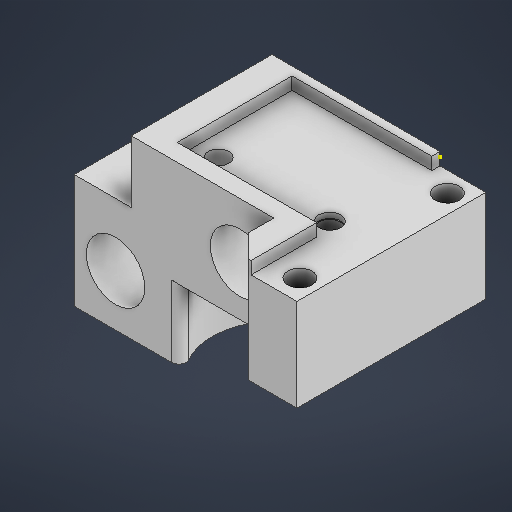
# Autodesk Inventor part: 固定传动
Saved by Autodesk Inventor 2025 (Build 290162000, 162)
## iProperties
Created: 2025-12-09
Part Number: 固定传动
Material: 常规
Document SubType Name: Modeling
Designer: XH
Density: 1 g/cm^3
Appearance: 默认
Author: XH
Autodesk Inventor part; units mm, degrees
ref_plane "YZ Plane" through (0, 0, 0) normal (1, 0, 0) x (0, 1, 0)
ref_plane "XZ Plane" through (0, 0, 0) normal (0, 1, 0) x (-1, 0, 0)
ref_plane "XY Plane" through (0, 0, 0) normal (0, 0, 1) x (1, 0, 0)
sketch "草图1" plane through (0, 0, 0) normal (0, 0, 1) x (1, 0, 0)
  line L0 (-22.2679, -12.5636) -> (3.7321, -12.5636) projected
  line L1 (-24.2679, 7.4364) -> (5.7321, 7.4364)
  line L2 (5.7321, 7.4364) -> (5.7321, -12.5636)
  line L3 (5.7321, -12.5636) -> (-24.2679, -12.5636)
  line L4 (-24.2679, -12.5636) -> (-24.2679, 7.4364)
  point P0 (-22.2679, -12.5636)
  point P1 (3.7321, -12.5636)
  dimension "d4" = 30
  dimension "d5" = 20
  constraints: 8 end point, 2 parallel, 1 collinear, 1 horizontal, 1 perpendicular
  measures "d4" distance of L1.start L1.end
  measures "d5" distance of L1.end L2.end
extrude "拉伸1" add sketch "草图1" along normal blind 19
sketch "草图2" plane through (0, 0, 0) normal (0, 0, -1) x (-1, 0, 0)
  line L0 (24.2679, 7.4364) -> (24.2679, -12.5636) projected
  line L1 (24.2679, -12.5636) -> (31.2679, -12.5636)
  line L2 (31.2679, -12.5636) -> (31.2679, -0.5636)
  line L3 (31.2679, -0.5636) -> (24.2679, -0.5636)
  line L4 (24.2679, -0.5636) -> (24.2679, -12.5636)
  point P0 (0, 0)
  dimension "d6" = 7
  dimension "d7" = 12
  constraints: 8 end point, 2 parallel, 1 horizontal, 1 perpendicular
  measures "d6" distance of L2.end L3.end
  measures "d7" distance of L1.end L2.end
extrude "拉伸2" add sketch "草图2" against normal up to surface (19 mm away)
sketch "草图3" plane through (0, 0, 0) normal (0, 0, -1) x (-1, 0, 0)
  circle A0 centre (-0.6256, 1.5535) radius 3
  circle A1 centre (26.4728, -5.3671) radius 4.1
  point P0 (0, 0)
  dimension "d10" = 6
  dimension "d11" = 8.2
  constraints: 2 centre point
  measures "d10" diameter of A0
  measures "d11" diameter of A1
extrude "拉伸3" cut sketch "草图3" against normal blind 40
sketch "草图4" plane through (5.7321, -12.5636, 0) normal (1, 0, 0) x (0, 0, -1)
  line L0 (-19, 0) -> (-4, 0)
  line L1 (-4, 0) -> (-4, 10)
  line L2 (-4, 10) -> (-19, 10)
  line L3 (-19, 10) -> (-19, 0)
  point P0 (0, 12.5636)
  dimension "d14" = 10
  dimension "d15" = 15
  constraints: 8 end point, 2 parallel, 1 horizontal, 1 perpendicular
  measures "d14" distance of L2.end L0.start
  measures "d15" distance of L1.end L2.end
extrude "拉伸4" cut sketch "草图4" against normal blind 21.75
chamfer "倒角1" distance 4 angle 45 1 edges at (-24.2679, -0.5636, 9.5)
sketch "草图5" plane through (5.7321, -12.5636, 0) normal (1, 0, 0) x (0, 0, -1)
  line L0 (-4, 0) -> (-19, 0) projected
  line L1 (-4, 0) -> (0, 0)
  line L2 (0, 0) -> (0, 10)
  line L3 (0, 10) -> (-4, 10)
  line L4 (-4, 10) -> (-4, 0)
  line L5 (0, 0) -> (0, 20) projected
  line L6 (-19, 10) -> (-4, 10) projected
  point P0 (0, 12.5636)
  constraints: 8 end point, 2 collinear, 2 parallel, 1 horizontal, 1 perpendicular
extrude "拉伸5" cut sketch "草图5" against normal blind 10
sketch "草图6" plane through (5.7321, -2.5636, 0) normal (0, -1, 0) x (1, 0, 0)
  line L0 (0, 0) -> (0, 19) projected
  line L1 (0, 0) -> (-8, 0)
  line L2 (-8, 0) -> (-8, 25.7509)
  line L3 (-8, 25.7509) -> (0, 25.7509)
  line L4 (0, 25.7509) -> (0, 0)
  line L5 (-12.3, 25.7509) -> (0, 25.7509) projected
  line L6 (-21.75, 19) -> (0, 19) projected
  line L7 (-8, 25.7509) -> (-10, 25.7509)
  line L8 (-10, 25.7509) -> (-10, 19)
  line L9 (-10, 19) -> (-8, 19)
  line L10 (-8, 19) -> (-8, 25.7509)
  point P0 (-5.7321, 0)
  point P1 (-8, 19)
  dimension "d23" = 8
  dimension "d28" = 10
  constraints: 16 end point, 4 parallel, 2 horizontal, 2 perpendicular, 1 collinear, 1 point on line
  measures "d23" distance between parallel lines of L2 L4
  measures "d28" distance between parallel lines of L4 L8
extrude "拉伸6" add sketch "草图6" against normal up to surface (10 mm away)
sketch "草图8" plane through (0, 0, 0) normal (0, 0, -1) x (-1, 0, 0)
  circle A0 centre (-0.6256, 1.5535) radius 3
  point P0 (0, 0)
  constraints: 1 centre point, 2 other
extrude "拉伸7" cut sketch "草图8" against normal blind 42.75
fillet "圆角1" radius 4 1 edges at (-4.2679, 2.4364, 19)
sketch "草图9" plane through (0, 0, 0) normal (0, 0, -1) x (-1, 0, 0)
  circle A0 centre (9.0791, 4.3462) radius 4.1
  point P0 (0, 0)
  dimension "d35" = 8.2
  constraints: 1 centre point, 1 other
  measures "d35" diameter of A0
extrude "拉伸8" cut sketch "草图9" against normal blind 33.75
delete faces "删除1" heal yes whole lump no faces at (-4.5364, 0.7697, 21.5592)
delete faces "删除2" heal yes whole lump no faces at (-1.434, 3.7348, 17.1673)
offset faces "大小1" outward 3 faces at (2.3988, 7.4364, 14.917) (-15.9384, 7.4364, 6.3333)
sketch "草图10" plane through (-16.0179, -2.5636, 19) normal (0, -1, 0) x (1, 0, 0)
  ellipse E0 centre (19.1097, 3.7017) end of major axis (18.1097, 3.7017) minor radius 1 projected
  ellipse E1 centre (19.1586, -16.9435) end of major axis (18.1586, -16.9435) minor radius 1 projected
  circle A0 centre (19.1097, 3.7017) radius 1.7
  circle A1 centre (19.1586, -16.9435) radius 1.7
  point P0 (16.0179, -19)
  dimension "d57" = 3.4
  dimension "d58" = 3.4
  constraints: 2 centre point, 2 coincident, 2 other
  measures "d57" diameter of A0
  measures "d58" diameter of A1
extrude "拉伸9" cut sketch "草图10" against normal blind 33.75 contours E0 | E1 | A0 | A1
offset faces "大小2" outward 1 faces at (-31.2679, -8.5636, 6.3333)
offset faces "大小3" outward 4 faces at (-30.9346, -0.5636, 6.3333)
sketch "草图11" plane through (-4.2679, -2.5636, 25.7509) normal (0, 0, 1) x (1, 0, 0)
  line L0 (10, 13) -> (-20, 13) projected
  line L1 (10, 13) -> (-20.4657, 13)
  line L2 (-20.4657, 13) -> (-20.4657, 12.2117)
  line L3 (-20.4657, 12.2117) -> (10, 12.2117)
  line L4 (10, 12.2117) -> (10, 13)
  line L5 (-8.462, 12.203) -> (17.6165, 12.2153)
  point P0 (4.2679, 2.5636)
  constraints: 10 end point, 2 parallel, 1 horizontal, 1 perpendicular, 1 point on line, 3 other
extrude "拉伸10" cut sketch "草图11" against normal blind 36.75
sketch "草图12" plane through (-16.0179, -12.5636, 4) normal (0, -1, 0) x (1, 0, 0)
  circle A0 centre (6.3087, 9) radius 8.2
  circle A1 centre (6.3087, 9) radius 9.2
  point P0 (16.0179, -4)
  dimension "d40" = 1
  constraints: 2 centre point, 2 other
  measures "d40" radial gap between concentric circles of A0 A1
extrude "拉伸11" cut sketch "草图12" against normal blind 10 contours A0 | A1
fillet "圆角2" radius 1 3 edges at (-16.6834, -7.5636, 19) (-16.0179, -7.5636, 6.3038) (-16.0179, -7.5636, 4)
chamfer "倒角2" distance 3.25 angle 45 1 edges at (-4.2679, 3.5422, 25.7509)
move faces "移动1" translate (0, 0, -0.75) faces at (-12.2629, -6.1847, 0)
sketch "草图14" plane through (-4.2679, -12.5636, -0.75) normal (0, 0, -1) x (-1, 0, 0)
  line L0 (0, 0) -> (28, 0) projected
  line L1 (3.0899, 0) -> (8.0899, 0)
  line L2 (8.0899, 0) -> (8.0899, 3.7894)
  line L3 (8.0899, 3.7894) -> (3.0899, 3.7894)
  line L4 (3.0899, 3.7894) -> (3.0899, 0)
  point P0 (-4.2679, 12.5636)
  point P1 (8.0899, 0)
  dimension "d51" = 5
  constraints: 8 end point, 2 parallel, 1 horizontal, 1 perpendicular, 1 point on line
  measures "d51" distance of L2.end L3.end
extrude "拉伸12" cut sketch "草图14" against normal blind 15.75
chamfer "倒角3" distance 2 angle 45 2 edges at (-7.3578, -8.7743, 1.625) (-12.3578, -8.7743, 1.625)
sketch "草图15" plane through (-24.2679, 9.6481, -0.75) normal (0, 1, 0) x (1, 0, 0)
  circle A0 centre (22.5841, -14.5011) radius 1.45
  circle A1 centre (7, -14.5011) radius 1.45
  line L0 (0, -19.75) -> (0, 0) projected
  point P0 (24.2679, -0.75)
  dimension "d63" = 2.9
  dimension "d64" = 2.9
  dimension "d65" = 15.5841
  dimension "d66" = 7
  constraints: 2 centre point, 1 horizontal alignment
  measures "d63" diameter of A0
  measures "d64" diameter of A1
  measures "d65" distance of A1.centre A0.centre
  measures "d66" distance from line of A1.centre L0
extrude "拉伸13" cut sketch "草图15" against normal blind 2.5
sketch "草图16" plane through (-24.2679, 9.6481, -0.75) normal (0, 1, 0) x (1, 0, 0)
  point P0 (24.2679, -0.75)
sketch "草图17" plane through (-24.2679, 9.6481, -0.75) normal (0, 1, 0) x (1, 0, 0)
  line L0 (13.2763, -13.5205) -> (16.2763, -13.513)
  line L1 (16.2763, -13.513) -> (16.2803, -15.113)
  line L2 (16.2803, -15.113) -> (13.2803, -15.1205)
  line L3 (13.2803, -15.1205) -> (13.2763, -13.5205) construction
  line L4 (4.1921, -1.3954) -> (25.2994, -1.3422)
  line L5 (25.2994, -1.3422) -> (25.339, -17.0902)
  line L6 (25.339, -17.0902) -> (4.2317, -17.1433)
  line L7 (4.2317, -17.1433) -> (4.1921, -1.3954)
  line L8 (3.6908, -0.8966) -> (25.7981, -0.841)
  line L9 (25.7981, -0.841) -> (25.8403, -17.5889)
  line L10 (25.8403, -17.5889) -> (3.733, -17.6446)
  line L11 (3.733, -17.6446) -> (3.6908, -0.8966)
  circle A0 centre (22.5575, -14.4619) radius 1.5557
  circle A1 centre (7, -14.5011) radius 1.45 projected
  point P0 (24.2679, -0.75)
  dimension "d67" = 0.5
  constraints: 24 end point, 1 centre point, 21 other
  measures "d67" distance between parallel lines of L7 L11
ref_plane "工作平面1" through (-15.3123, 10.3965, 10.8693) normal (0, -1, 0) x (0.9999968, 0, -0.0025167)
extrude "拉伸14" add sketch "草图17" along normal up to surface (0.7484 mm away) contours L4 L5 L6 L7
sketch "草图18" plane through (-24.2679, 9.6481, -0.75) normal (0, 1, 0) x (1, 0, 0)
  line L0 (25.339, -17.0902) -> (4.2317, -17.1433) projected
  line L1 (4.2317, -17.1433) -> (4.1921, -1.3954) projected
  line L2 (4.1921, -1.3954) -> (25.2994, -1.3422) projected
  line L3 (25.2994, -1.3422) -> (25.339, -17.0902) projected
  circle A0 centre (27.3597, -23.4517) radius 1.7 projected
  circle A1 centre (27.4086, -2.8065) radius 1.7 projected
  line L4 (23.25, -26.5009) -> (20, -23.2509) projected
  line L5 (30, -26.5009) -> (23.25, -26.5009) projected
  line L6 (30, 0) -> (30, -26.5009) projected
  line L7 (0, 0) -> (30, 0) projected
  line L8 (0, -19.75) -> (0, 0) projected
  line L9 (20, -19.75) -> (0, -19.75) projected
  line L10 (20, -23.2509) -> (20, -19.75) projected
  line L11 (3.9916, -1.1959) -> (4.0322, -17.3438)
  line L12 (4.0322, -17.3438) -> (25.5395, -17.2897)
  line L13 (25.5395, -17.2897) -> (25.4989, -1.1417)
  line L14 (25.4989, -1.1417) -> (3.9916, -1.1959)
  point P0 (24.2679, -0.75)
  dimension "d70" = 0.2
  constraints: 8 end point, 3 other
  measures "d70" distance between parallel lines of L1 L11
extrude "拉伸15" add sketch "草图18" along normal blind 2.5 contours L4 L10 L9 L8 L7 L6 L5
sketch "草图19" plane through (-24.2679, 12.1481, -0.75) normal (0, 1, 0) x (1, 0, 0)
  point P0 (24.2679, -0.75)
sketch "草图21" plane through (-20.2357, 9.6481, 16.5938) normal (0, 1, 0) x (0.9999968, 0, -0.0025167)
  line L0 (0, 16.148) -> (0, 0) projected
  line L1 (0, 0) -> (21.5074, 0) projected
  line L2 (21.5074, 0) -> (21.5074, 16.148) projected
  line L3 (21.5074, 16.148) -> (0, 16.148) projected
  line L4 (21.3074, 0.2) -> (0.2, 0.2) projected
  line L5 (0.2, 0.2) -> (0.2, 15.948) projected
  line L6 (0.2, 15.948) -> (21.3074, 15.948) projected
  line L7 (21.3074, 15.948) -> (21.3074, 0.2) projected
  point P0 (20.2774, 16.5428)
extrude "拉伸16" add sketch "草图21" along normal up to surface (0.7484 mm away)
sketch "草图22" plane through (-24.2679, 12.1481, -0.75) normal (0, 1, 0) x (1, 0, 0)
  line L0 (30, 0) -> (20, 0) projected
  line L1 (30, 0) -> (23.5601, 0)
  line L2 (23.5601, 0) -> (23.5601, -28.4303)
  line L3 (23.5601, -28.4303) -> (30, -28.4303)
  line L4 (30, -28.4303) -> (30, 0)
  point P0 (24.2679, -0.75)
  constraints: 8 end point, 2 parallel, 1 horizontal, 1 perpendicular, 1 point on line
extrude "拉伸17" cut sketch "草图22" against normal up to surface (1.7516 mm away)
